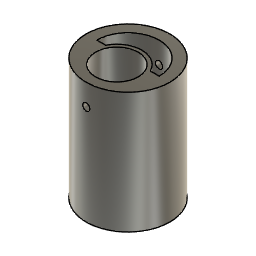
Motor Sleeve v9 (Autodesk Fusion 360 design; units mm, degrees)
Autodesk Fusion 360 part; units mm, degrees
sketch "Sketch8" plane through (0, 0, 0) normal (0, 0, 1) x (1, 0, 0)
  circle A0 centre (0, 0) radius 37.3062
  circle A1 centre (0, 0) radius 27.7812
  dimension "d25" = 74.6125
  dimension "d26" = 55.5625
  constraint coincident A0.centre A1.centre
  constraint concentric A0 A1
  measures "d25" diameter of A0
  measures "d26" diameter of A1
extrude "Extrude4" add sketch "Sketch8" along normal blind 50.8
sketch "Sketch9" plane through (0, 0, 50.8) normal (0, 0, 1) x (-1, 0, 0)
  circle A0 centre (0, 0) radius 27.7812
  circle A1 centre (0, 0) radius 37.3062
  circle A2 centre (0, 0) radius 37.3062
  circle A3 centre (0, 0) radius 9.9219
  line L0 (0, 0) -> (-27.7812, 0)
  line L1 (0, 0) -> (27.7812, 0)
  dimension "d29" = 19.8438
  constraint coincident A0.centre A1.centre
  constraint concentric A2 A3
  constraint coincident A0 L0.end
  constraint horizontal L0
  constraint coincident A0 L1.end
  constraint parallel L0 L1
  measures "d29" diameter of A3
extrude "Extrude5" add sketch "Sketch9" along normal blind 6.35 contours A0 A3 L0 L1 | A1 A2 picked at (-14.6242, 16.1245)
sketch "Sketch10" plane through (0, 0, 57.15) normal (0, 0, 1) x (-1, 0, 0)
  arc A0 (9.9219, 0) -> (-9.9219, 0) centre (0, 0) ccw
  line L0 (9.9219, 0) -> (27.7812, 0)
  arc A1 (-27.7812, 0) -> (27.7812, 0) centre (0, 0) ccw
  line L1 (-27.7812, 0) -> (-9.9219, 0)
  circle A2 centre (0, 0) radius 37.3062
  line L2 (0, 0) -> (0, 9.9219)
  circle A3 centre (0, 9.9219) radius 19.05
  circle A4 centre (0, 9.9219) radius 22.225
  circle A5 centre (0, 0) radius 32.1469
  circle A6 centre (0, 0) radius 37.3062
  circle A7 centre (0, 0) radius 27.7812
  line L3 (27.7812, 0) -> (19.8874, 0)
  line L4 (-19.8874, 0) -> (-27.7812, 0)
  dimension "d32" = 38.1
  dimension "d33" = 44.45
  constraint coincident A0.centre A1.centre
  constraint midpoint A0 L2.end
  constraint coincident L2.end A3.centre
  constraint concentric A3 A4
  constraint tangent A4 A5
  constraint concentric A5 A6
  constraint concentric A6 A7
  constraint coincident L0.end A1.end
  constraint coincident A4 L3.end
  constraint coincident L0 L3.end
  constraint coincident A4 L4.start
  constraint coincident L1 L4.start
  constraint coincident A1.start L1.start
  measures "d32" diameter of A3
  measures "d33" diameter of A4
extrude "Extrude6" add sketch "Sketch10" along normal blind 50.8 contours L0 A3 A4 A7 | L0 L1 A3 A4 | L0 A4 A7 L3 | L1 A3 A4 A7 | A5 | L1 A4 A7 L4 | A3 A4 A7 | A2 A6
ref_plane "WorkPlane1" through (0, -38.1, 0) normal (0, 1, 0) x (0, 0, 1)
sketch "Sketch11" plane through (0, -38.1, 0) normal (0, 1, 0) x (1, 0, 0)
  line L0 (0, 0) -> (0, -88.9)
  circle A0 centre (0, -88.9) radius 3.175
  dimension "d37" = 6.35
  constraint coincident L0.start origin
  constraint vertical L0
  constraint coincident L0.end A0.centre
  measures "d37" diameter of A0
hole "Hole2" at (0, -38.1, 88.9) direction (0, 1, 0) diameter 6.35 depth 15.24 tip angle 118
ref_plane "WorkPlane2" through (0, 38.1, 0) normal (0, 1, 0) x (0, 0, 1)
sketch "Sketch12" plane through (0, 38.1, 0) normal (0, 1, 0) x (1, 0, 0)
  line L0 (0, 0) -> (0, -88.9)
  circle A0 centre (0, -88.9) radius 3.175
  line L1 (0, -88.9) -> (0, -107.95)
  dimension "d42" = 88.9
  dimension "d43" = 6.35
  dimension "d47" = 19.05
  constraint vertical L0
  constraint coincident L0.start origin
  constraint coincident L0.end A0.centre
  constraint parallel L0 L1
  measures "d42" distance of L0.start L0.end
  measures "d43" diameter of A0
  measures "d47" distance of L0.end L1.end
hole "Hole3" at (0, 38.1, 88.9) direction (0, -1, 0) diameter 6.35 depth 15.24 tip angle 118
sketch "Sketch7" plane through (0, 0, 0) normal (0, 0, 1) x (1, 0, 0)
equation "d25 = 3 in - ( ( 1 / 16 ) * 1 in )"
equation "d26 = 3 in - ( ( 1 / 16 ) * 1 in ) - ( ( 3 / 4 ) * 1 in )"
equation "d29 = ( ( 3 / 4 ) * 1 in ) + ( 1 / 32 ) * 1 in"
equation "d33 = 1.5 in + ( ( 1 / 4 ) * 1 in )"
